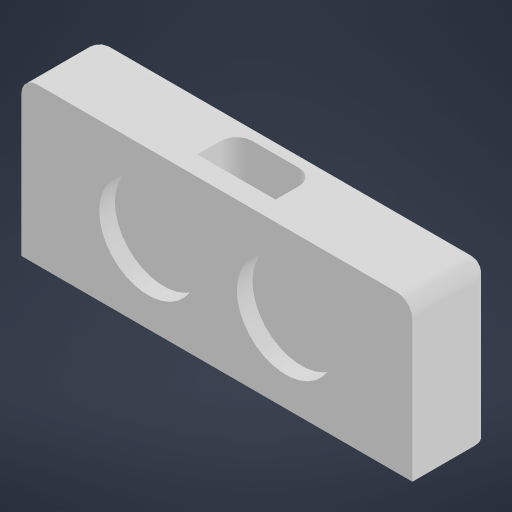
# Autodesk Inventor part: A1 Holder
Saved by Autodesk Inventor 2024.1 (Build 281209000, 209)
## iProperties
Created: 2023-09-11
Part Number: A1 Holder
Material: Generic
Document SubType Name: Modeling
Designer: User
Density: 1 g/cm^3
Appearance: Default
Author: User
Autodesk Inventor part; units mm, degrees
ref_plane "YZ Plane" through (0, 0, 0) normal (1, 0, 0) x (0, 1, 0)
ref_plane "XZ Plane" through (0, 0, 0) normal (0, 1, 0) x (-1, 0, 0)
ref_plane "XY Plane" through (0, 0, 0) normal (0, 0, 1) x (1, 0, 0)
sketch "Sketch6" plane through (0, 0, 0) normal (0, 0, 1) x (1, 0, 0)
  line L0 (0, 0) -> (-50, 0)
  line L1 (-50, 0) -> (-50, 20)
  line L2 (-50, 20) -> (0, 20)
  line L3 (0, 20) -> (0, 0)
  dimension "d55" = 50
  dimension "d56" = 20
  constraints: 8 end point, 2 parallel, 1 horizontal, 1 perpendicular
  measures "d55" distance of L1.end L2.end
  measures "d56" distance of L0.end L1.end
extrude "Extrusion5" add sketch "Sketch6" along normal blind 10
sketch "Sketch7" plane through (0, 0, 10) normal (0, 0, 1) x (1, 0, 0)
  circle A0 centre (-33.8, 10) radius 6.25
  circle A1 centre (-16.2, 10) radius 6.25
  point P0 (0, 0)
  dimension "d59" = 12.5
  dimension "d60" = 12.5
  constraints: 2 centre point
  measures "d59" diameter of A0
  measures "d60" diameter of A1
extrude "Extrusion6" cut sketch "Sketch7" against normal blind 2
sketch "Sketch8" plane through (-50, 20, 0) normal (0, 1, 0) x (1, 0, 0)
  line L0 (50, 0) -> (30, 0)
  line L1 (30, 0) -> (30, -2.5)
  line L2 (30, -2.5) -> (50, -2.5)
  line L3 (50, -2.5) -> (50, 0)
  line L4 (30, -2.5) -> (20, -2.5)
  line L5 (20, -2.5) -> (20, -7.5)
  line L6 (20, -7.5) -> (30, -7.5)
  line L7 (30, -7.5) -> (30, -2.5)
  dimension "d63" = 20
  dimension "d64" = 2.5
  dimension "d65" = 10
  dimension "d66" = 5
  constraints: 16 end point, 4 parallel, 2 horizontal, 2 perpendicular
  measures "d63" distance of L2.end L1.end
  measures "d64" distance of L1.end L0.end
  measures "d65" distance of L6.end L5.end
  measures "d66" distance of L5.end L4.end
extrude "Extrusion7" cut sketch "Sketch8" against normal blind 10 contours L7 L6 L5 L4
fillet "Fillet4" radius 2 2 edges at (-30, 15, 2.5) (-20, 15, 2.5)
fillet "Fillet5" radius 2 5 edges at (0, 20, 5) (-50, 20, 5) (-50, 10, 0) (-25, 20, 0) (0, 10, 0)
body "Solid2"
